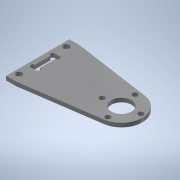
# Autodesk Inventor part: Shoulder_side_frame
Saved by Autodesk Inventor 2020.4 (Build 244396000, 396)
## iProperties
Created: 2016-05-05
Part Number: Shoulder_side_frame
Material: アルミニウム 2014-T4
Document SubType Name: Modeling
Designer: hiroaki
Density: 2.8 g/cm^3
Appearance: 滑らか - 淡い灰色
Mass: 5.10167 g
Surface Area: 23.2279 cm^2
Volume: 1.82202 cm^3
Description: A2017 T2
Author: hiroaki
Autodesk Inventor part; units mm, degrees
ref_plane "YZ Plane" through (0, 0, 0) normal (1, 0, 0) x (0, 1, 0)
ref_plane "XZ Plane" through (0, 0, 0) normal (0, 1, 0) x (-1, 0, 0)
ref_plane "XY Plane" through (0, 0, 0) normal (0, 0, 1) x (1, 0, 0)
sketch "スケッチ1" plane through (0, 0, 0) normal (0, 0, 1) x (1, 0, 0)
  circle A0 centre (-1.476, 8.3709) radius 1.35
  circle A1 centre (0, 0) radius 5.05
  line L0 (-39.8, 6) -> (-37.3, 6) construction
  line L1 (-37.3, 6) -> (-37.3, -6) construction
  line L2 (-37.3, -6) -> (-39.8, -6) construction
  line L3 (-39.8, -6) -> (-39.8, 6) construction
  line L4 (-37.25, 6.05) -> (-39.85, 6.05) construction
  line L5 (-39.85, 6.05) -> (-39.85, -6.05) construction
  line L6 (-39.85, -6.05) -> (-37.25, -6.05) construction
  line L7 (-37.25, -6.05) -> (-37.25, 6.05) construction
  circle A2 centre (-39.85, 5) radius 1.05 construction
  line L8 (-37.25, 6.05) -> (-39.85, 6.05)
  arc A3 (-39.85, 6.05) -> (-39.85, 3.95) centre (-39.85, 5) ccw
  line L9 (-39.85, 3.95) -> (-39.85, -3.95)
  line L10 (-38.55, 6.05) -> (-38.55, -6.05) construction
  line L11 (-39.85, 0) -> (-37.3, 0) construction
  arc A4 (-39.85, -3.95) -> (-39.85, -6.05) centre (-39.85, -5) ccw
  line L12 (-39.85, -6.05) -> (-37.25, -6.05)
  line L13 (-37.25, 3.95) -> (-37.25, -3.95)
  arc A5 (-37.25, 3.95) -> (-37.25, 6.05) centre (-37.25, 5) ccw
  arc A6 (-37.25, -6.05) -> (-37.25, -3.95) centre (-37.25, -5) ccw
  circle A7 centre (-39.8, 12) radius 1.55
  circle A8 centre (-39.8, -12) radius 1.55
  line L14 (-42.3, 16) -> (-37.3, 16)
  line L15 (-42.3, -16) -> (-37.3, -16)
  arc A9 (1.5019, -10.392) -> (1.5019, 10.392) centre (0, 0) ccw
  line L16 (-42.3, 16) -> (-42.3, -16)
  line L17 (-37.3, 16) -> (1.5019, 10.392)
  line L18 (1.5019, -10.392) -> (-37.3, -16)
  line L19 (-1.476, 8.3709) -> (0, 0) construction
  line L20 (0, 10.6091) -> (0, -10.6091) construction
  circle A10 centre (-8.3709, -1.476) radius 1.35
  circle A11 centre (1.476, -8.3709) radius 1.35
  circle A12 centre (8.3709, 1.476) radius 1.35
  point P0 (-38.575, 0)
  dimension "d29" = 2.1
  dimension "d4" = 2.7
  dimension "d9" = 10.1
  dimension "d10" = 2.5
  dimension "d30" = 0.05
  dimension "d31" = 6
  dimension "d33" = 3.1
  dimension "d57" = 32
  dimension "d61" = 42.3
  dimension "d62" = 5
  dimension "d63" = 2.5
  dimension "d65" = 10
  dimension "d66" = 10.5
  dimension "d67" = 8.5
  dimension "d69" = 10
  dimension "d72" = 360
  constraints: 42 end point, 12 centre point, 10 point on circle, 6 midpoint, 5 parallel, 5 symmetric about line, 5 tangent, 4 coincident, 4 perpendicular, 3 horizontal, 3 point on line, 3 vertical, 3 vertical alignment, 2 collinear, 2 equal radius, 1 horizontal alignment, 16 other
  measures "d4" diameter of A0
  measures "d9" diameter of A1
  measures "d10" distance of L0.start L0.end
  measures "d30" distance between parallel lines of L4 L0
  measures "d31" distance from line of L0 A7.centre
  measures "d33" diameter of A7
  measures "d57" distance of L15.start L14.start
  measures "d61" distance from line of point (0, 0) L16
  measures "d62" distance of L14.start L14.end
  measures "d63" horizontal distance of L14.start A7.centre
  measures "d65" distance between parallel lines of L14 L0
  measures "d66" radius of A9
  measures "d67" distance of L19.start L19.end
  measures "d69" angle of L20 L19
extrude "押し出し1" add sketch "スケッチ1" along normal blind 2
equation "\"d23\" = 7"
